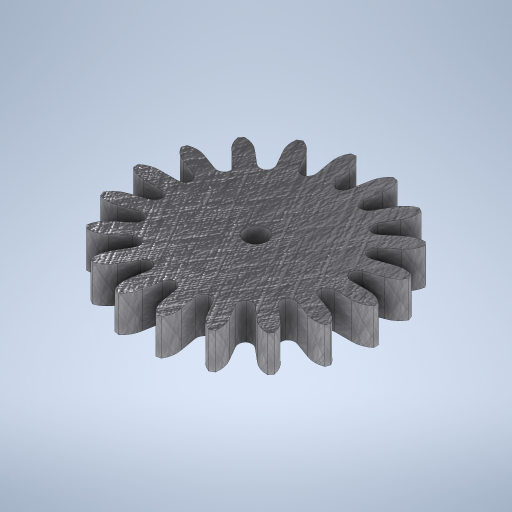
# Autodesk Inventor part: Rear_motor
Saved by Autodesk Inventor 2024 (Build 280153020, 153B)
## iProperties
Created: 2023-05-21
Part Number: Rear_motor
Material: Generic
Document SubType Name: Modeling
Designer: Diego
Density: 1 g/cm^3
Appearance: Default
Author: Diego
Autodesk Inventor part; units mm, degrees
ref_plane "YZ Plane" through (0, 0, 0) normal (1, 0, 0) x (0, 1, 0)
ref_plane "XZ Plane" through (0, 0, 0) normal (0, 1, 0) x (-1, 0, 0)
ref_plane "XY Plane" through (0, 0, 0) normal (0, 0, 1) x (1, 0, 0)
sketch "Sketch1" plane through (0, 0, 0) normal (0, 1, 0) x (-1, 0, 0)
  circle A0 centre (0, 0) radius 1.4
  arc A1 (14.997, -0.3) -> (14.997, 0.3) centre (0, 0) ccw
  line L0 (0, 0) -> (19.0442, 1.4988) construction
  line L1 (0, 0) -> (19.3478, 0) construction
  line L2 (0, 0) -> (18.7398, -1.4749) construction
  arc A2 (14.997, 0.3) -> (12.9599, 1.02) centre (13.0458, -1.9788) ccw
  arc A3 (12.9599, -1.02) -> (14.997, -0.3) centre (13.0458, 1.9788) ccw
  line L3 (12.9599, 1.02) -> (10.8129, 1.02)
  line L4 (12.9599, -1.02) -> (10.8129, -1.02)
  arc A4 (10.8129, -1.02) -> (9.8299, -1.8363) centre (10.8129, -2.02) ccw
  arc A5 (9.8299, 1.8363) -> (10.8129, 1.02) centre (10.8129, 2.02) ccw
  line L5 (12.5272, 3.4741) -> (10.5097, 2.7398)
  arc A6 (10.5097, 2.7398) -> (9.8652, 1.6364) centre (10.8517, 1.8001) ccw
  arc A7 (8.6091, 5.0876) -> (9.812, 4.6567) centre (9.47, 5.5964) ccw
  arc A8 (13.99, 5.4112) -> (11.8295, 5.391) centre (12.9359, 2.6025) ccw
  line L6 (11.8295, 5.391) -> (9.812, 4.6567)
  arc A9 (14.1952, 4.8474) -> (13.99, 5.4112) centre (0, 0) ccw
  arc A10 (12.5272, 3.4741) -> (14.1952, 4.8474) centre (11.5823, 6.3214) ccw
  line L7 (10.5835, 7.5491) -> (8.9388, 6.1691)
  arc A11 (8.9388, 6.1691) -> (8.7106, 4.9119) centre (9.5816, 5.403) ccw
  arc A12 (6.3498, 7.7253) -> (7.6276, 7.7318) centre (6.9848, 8.4978) ccw
  arc A13 (11.2955, 9.8697) -> (9.2723, 9.1118) centre (11.2656, 6.8698) ccw
  line L8 (9.2723, 9.1118) -> (7.6276, 7.7318)
  arc A14 (11.6812, 9.4101) -> (11.2955, 9.8697) centre (0, 0) ccw
  arc A15 (10.5835, 7.5491) -> (11.6812, 9.4101) centre (8.7217, 9.9015) ccw
  line L9 (7.3633, 10.7136) -> (6.2898, 8.8543)
  arc A16 (6.2898, 8.8543) -> (6.5053, 7.5948) centre (7.1558, 8.3543) ccw
  arc A17 (3.3247, 9.4312) -> (4.5232, 9.8743) centre (3.6571, 10.3743) ccw
  arc A18 (7.2387, 13.1378) -> (5.5966, 11.7336) centre (8.2366, 10.3086) ccw
  line L10 (5.5966, 11.7336) -> (4.5232, 9.8743)
  arc A19 (7.7583, 12.8378) -> (7.2387, 13.1378) centre (0, 0) ccw
  arc A20 (7.3633, 10.7136) -> (7.7583, 12.8378) centre (4.8092, 12.2874) ccw
  line L11 (3.2549, 12.5859) -> (2.8821, 10.4716)
  arc A21 (2.8821, 10.4716) -> (3.5154, 9.3617) centre (3.8669, 10.2979) ccw
  arc A22 (-0.1015, 9.9995) -> (0.8732, 10.8258) centre (-0.1116, 10.9994) ccw
  arc A23 (2.3088, 14.8213) -> (1.246, 12.9402) centre (4.2141, 12.504) ccw
  line L12 (1.246, 12.9402) -> (0.8732, 10.8258)
  arc A24 (2.8996, 14.7171) -> (2.3088, 14.8213) centre (0, 0) ccw
  arc A25 (3.2549, 12.5859) -> (2.8996, 14.7171) centre (0.3166, 13.1912) ccw
  line L13 (-1.246, 12.9402) -> (-0.8732, 10.8258)
  arc A26 (-0.8732, 10.8258) -> (0.1015, 9.9995) centre (0.1116, 10.9994) ccw
  arc A27 (-3.5154, 9.3617) -> (-2.8821, 10.4716) centre (-3.8669, 10.2979) ccw
  arc A28 (-2.8996, 14.7171) -> (-3.2549, 12.5859) centre (-0.3166, 13.1912) ccw
  line L14 (-3.2549, 12.5859) -> (-2.8821, 10.4716)
  arc A29 (-2.3088, 14.8213) -> (-2.8996, 14.7171) centre (0, 0) ccw
  arc A30 (-1.246, 12.9402) -> (-2.3088, 14.8213) centre (-4.2141, 12.504) ccw
  line L15 (-5.5966, 11.7336) -> (-4.5232, 9.8743)
  arc A31 (-4.5232, 9.8743) -> (-3.3247, 9.4312) centre (-3.6571, 10.3743) ccw
  arc A32 (-6.5053, 7.5948) -> (-6.2898, 8.8543) centre (-7.1558, 8.3543) ccw
  arc A33 (-7.7583, 12.8378) -> (-7.3633, 10.7136) centre (-4.8092, 12.2874) ccw
  line L16 (-7.3633, 10.7136) -> (-6.2898, 8.8543)
  arc A34 (-7.2387, 13.1378) -> (-7.7583, 12.8378) centre (0, 0) ccw
  arc A35 (-5.5966, 11.7336) -> (-7.2387, 13.1378) centre (-8.2366, 10.3086) ccw
  line L17 (-9.2723, 9.1118) -> (-7.6276, 7.7318)
  arc A36 (-7.6276, 7.7318) -> (-6.3498, 7.7253) centre (-6.9848, 8.4978) ccw
  arc A37 (-8.7106, 4.9119) -> (-8.9388, 6.1691) centre (-9.5816, 5.403) ccw
  arc A38 (-11.6812, 9.4101) -> (-10.5835, 7.5491) centre (-8.7217, 9.9015) ccw
  line L18 (-10.5835, 7.5491) -> (-8.9388, 6.1691)
  arc A39 (-11.2955, 9.8697) -> (-11.6812, 9.4101) centre (0, 0) ccw
  arc A40 (-9.2723, 9.1118) -> (-11.2955, 9.8697) centre (-11.2656, 6.8698) ccw
  line L19 (-11.8295, 5.391) -> (-9.812, 4.6567)
  arc A41 (-9.812, 4.6567) -> (-8.6091, 5.0876) centre (-9.47, 5.5964) ccw
  arc A42 (-9.8652, 1.6364) -> (-10.5097, 2.7398) centre (-10.8517, 1.8001) ccw
  arc A43 (-14.1952, 4.8474) -> (-12.5272, 3.4741) centre (-11.5823, 6.3214) ccw
  line L20 (-12.5272, 3.4741) -> (-10.5097, 2.7398)
  arc A44 (-13.99, 5.4112) -> (-14.1952, 4.8474) centre (0, 0) ccw
  arc A45 (-11.8295, 5.391) -> (-13.99, 5.4112) centre (-12.9359, 2.6025) ccw
  line L21 (-12.9599, 1.02) -> (-10.8129, 1.02)
  arc A46 (-10.8129, 1.02) -> (-9.8299, 1.8363) centre (-10.8129, 2.02) ccw
  arc A47 (-9.8299, -1.8363) -> (-10.8129, -1.02) centre (-10.8129, -2.02) ccw
  arc A48 (-14.997, -0.3) -> (-12.9599, -1.02) centre (-13.0458, 1.9788) ccw
  line L22 (-12.9599, -1.02) -> (-10.8129, -1.02)
  arc A49 (-14.997, 0.3) -> (-14.997, -0.3) centre (0, 0) ccw
  arc A50 (-12.9599, 1.02) -> (-14.997, 0.3) centre (-13.0458, -1.9788) ccw
  line L23 (-12.5272, -3.4741) -> (-10.5097, -2.7398)
  arc A51 (-10.5097, -2.7398) -> (-9.8652, -1.6364) centre (-10.8517, -1.8001) ccw
  arc A52 (-8.6091, -5.0876) -> (-9.812, -4.6567) centre (-9.47, -5.5964) ccw
  arc A53 (-13.99, -5.4112) -> (-11.8295, -5.391) centre (-12.9359, -2.6025) ccw
  line L24 (-11.8295, -5.391) -> (-9.812, -4.6567)
  arc A54 (-14.1952, -4.8474) -> (-13.99, -5.4112) centre (0, 0) ccw
  arc A55 (-12.5272, -3.4741) -> (-14.1952, -4.8474) centre (-11.5823, -6.3214) ccw
  line L25 (-10.5835, -7.5491) -> (-8.9388, -6.1691)
  arc A56 (-8.9388, -6.1691) -> (-8.7106, -4.9119) centre (-9.5816, -5.403) ccw
  arc A57 (-6.3498, -7.7253) -> (-7.6276, -7.7318) centre (-6.9848, -8.4978) ccw
  arc A58 (-11.2955, -9.8697) -> (-9.2723, -9.1118) centre (-11.2656, -6.8698) ccw
  line L26 (-9.2723, -9.1118) -> (-7.6276, -7.7318)
  arc A59 (-11.6812, -9.4101) -> (-11.2955, -9.8697) centre (0, 0) ccw
  arc A60 (-10.5835, -7.5491) -> (-11.6812, -9.4101) centre (-8.7217, -9.9015) ccw
  line L27 (-7.3633, -10.7136) -> (-6.2898, -8.8543)
  arc A61 (-6.2898, -8.8543) -> (-6.5053, -7.5948) centre (-7.1558, -8.3543) ccw
  arc A62 (-3.3247, -9.4312) -> (-4.5232, -9.8743) centre (-3.6571, -10.3743) ccw
  arc A63 (-7.2387, -13.1378) -> (-5.5966, -11.7336) centre (-8.2366, -10.3086) ccw
  line L28 (-5.5966, -11.7336) -> (-4.5232, -9.8743)
  arc A64 (-7.7583, -12.8378) -> (-7.2387, -13.1378) centre (0, 0) ccw
  arc A65 (-7.3633, -10.7136) -> (-7.7583, -12.8378) centre (-4.8092, -12.2874) ccw
  line L29 (-3.2549, -12.5859) -> (-2.8821, -10.4716)
  arc A66 (-2.8821, -10.4716) -> (-3.5154, -9.3617) centre (-3.8669, -10.2979) ccw
  arc A67 (0.1015, -9.9995) -> (-0.8732, -10.8258) centre (0.1116, -10.9994) ccw
  arc A68 (-2.3088, -14.8213) -> (-1.246, -12.9402) centre (-4.2141, -12.504) ccw
  line L30 (-1.246, -12.9402) -> (-0.8732, -10.8258)
  arc A69 (-2.8996, -14.7171) -> (-2.3088, -14.8213) centre (0, 0) ccw
  arc A70 (-3.2549, -12.5859) -> (-2.8996, -14.7171) centre (-0.3166, -13.1912) ccw
  line L31 (1.246, -12.9402) -> (0.8732, -10.8258)
  arc A71 (0.8732, -10.8258) -> (-0.1015, -9.9995) centre (-0.1116, -10.9994) ccw
  arc A72 (3.5154, -9.3617) -> (2.8821, -10.4716) centre (3.8669, -10.2979) ccw
  arc A73 (2.8996, -14.7171) -> (3.2549, -12.5859) centre (0.3166, -13.1912) ccw
  line L32 (3.2549, -12.5859) -> (2.8821, -10.4716)
  arc A74 (2.3088, -14.8213) -> (2.8996, -14.7171) centre (0, 0) ccw
  arc A75 (1.246, -12.9402) -> (2.3088, -14.8213) centre (4.2141, -12.504) ccw
  line L33 (5.5966, -11.7336) -> (4.5232, -9.8743)
  arc A76 (4.5232, -9.8743) -> (3.3247, -9.4312) centre (3.6571, -10.3743) ccw
  arc A77 (6.5053, -7.5948) -> (6.2898, -8.8543) centre (7.1558, -8.3543) ccw
  arc A78 (7.7583, -12.8378) -> (7.3633, -10.7136) centre (4.8092, -12.2874) ccw
  line L34 (7.3633, -10.7136) -> (6.2898, -8.8543)
  arc A79 (7.2387, -13.1378) -> (7.7583, -12.8378) centre (0, 0) ccw
  arc A80 (5.5966, -11.7336) -> (7.2387, -13.1378) centre (8.2366, -10.3086) ccw
  line L35 (9.2723, -9.1118) -> (7.6276, -7.7318)
  arc A81 (7.6276, -7.7318) -> (6.3498, -7.7253) centre (6.9848, -8.4978) ccw
  arc A82 (8.7106, -4.9119) -> (8.9388, -6.1691) centre (9.5816, -5.403) ccw
  arc A83 (11.6812, -9.4101) -> (10.5835, -7.5491) centre (8.7217, -9.9015) ccw
  line L36 (10.5835, -7.5491) -> (8.9388, -6.1691)
  arc A84 (11.2955, -9.8697) -> (11.6812, -9.4101) centre (0, 0) ccw
  arc A85 (9.2723, -9.1118) -> (11.2955, -9.8697) centre (11.2656, -6.8698) ccw
  line L37 (11.8295, -5.391) -> (9.812, -4.6567)
  arc A86 (9.812, -4.6567) -> (8.6091, -5.0876) centre (9.47, -5.5964) ccw
  arc A87 (9.8652, -1.6364) -> (10.5097, -2.7398) centre (10.8517, -1.8001) ccw
  arc A88 (14.1952, -4.8474) -> (12.5272, -3.4741) centre (11.5823, -6.3214) ccw
  line L38 (12.5272, -3.4741) -> (10.5097, -2.7398)
  arc A89 (13.99, -5.4112) -> (14.1952, -4.8474) centre (0, 0) ccw
  arc A90 (11.8295, -5.391) -> (13.99, -5.4112) centre (12.9359, -2.6025) ccw
  arc A91 (8.7106, 4.9119) -> (8.6091, 5.0876) centre (0, 0) ccw
  arc A92 (6.5053, 7.5948) -> (6.3498, 7.7253) centre (0, 0) ccw
  arc A93 (3.5154, 9.3617) -> (3.3247, 9.4312) centre (0, 0) ccw
  arc A94 (0.1015, 9.9995) -> (-0.1015, 9.9995) centre (0, 0) ccw
  arc A95 (-3.3247, 9.4312) -> (-3.5154, 9.3617) centre (0, 0) ccw
  arc A96 (-6.3498, 7.7253) -> (-6.5053, 7.5948) centre (0, 0) ccw
  arc A97 (-8.6091, 5.0876) -> (-8.7106, 4.9119) centre (0, 0) ccw
  arc A98 (-9.8299, 1.8363) -> (-9.8652, 1.6364) centre (0, 0) ccw
  arc A99 (-9.8652, -1.6364) -> (-9.8299, -1.8363) centre (0, 0) ccw
  arc A100 (-8.7106, -4.9119) -> (-8.6091, -5.0876) centre (0, 0) ccw
  arc A101 (-6.5053, -7.5948) -> (-6.3498, -7.7253) centre (0, 0) ccw
  arc A102 (-3.5154, -9.3617) -> (-3.3247, -9.4312) centre (0, 0) ccw
  arc A103 (-0.1015, -9.9995) -> (0.1015, -9.9995) centre (0, 0) ccw
  arc A104 (3.3247, -9.4312) -> (3.5154, -9.3617) centre (0, 0) ccw
  arc A105 (6.3498, -7.7253) -> (6.5053, -7.5948) centre (0, 0) ccw
  arc A106 (8.6091, -5.0876) -> (8.7106, -4.9119) centre (0, 0) ccw
  circle A107 centre (0, 0) radius 10 construction
  circle A108 centre (0, 0) radius 13.0054 construction
  circle A109 centre (0, 0) radius 15 construction
  point P0 (9.9478, -1.02)
  point P1 (9.9478, 1.02)
  point P2 (9.8537, 1.7375)
  point P3 (8.6652, 5.0028)
  point P4 (6.4315, 7.6648)
  point P5 (3.4221, 9.4023)
  point P6 (0, 10.0057)
  point P7 (-3.4221, 9.4023)
  point P8 (-6.4315, 7.6648)
  point P9 (-8.6652, 5.0028)
  point P10 (-9.8537, 1.7375)
  point P11 (-9.8537, -1.7375)
  point P12 (-8.6652, -5.0028)
  point P13 (-6.4315, -7.6648)
  point P14 (-3.4221, -9.4023)
  point P15 (0, -10.0057)
  point P16 (3.4221, -9.4023)
  point P17 (6.4315, -7.6648)
  point P18 (8.6652, -5.0028)
  point P19 (9.8537, -1.7375)
  dimension "d0" = 2.8
  dimension "d4" = 9
  dimension "d5" = 4.5
  dimension "d6" = 3
  dimension "d7" = 0.3
  dimension "d8" = 0.6
  dimension "d9" = 3
  dimension "d11" = 1
  dimension "d12" = 1
  dimension "d15" = 360
  dimension "d19" = 20
  constraints: 212 point on circle, 110 centre point, 78 end point, 5 coincident, 4 point on line, 3 horizontal, 2 tangent, 361 other
  measures "d0" diameter of A0
  measures "d4" angle of L2 L0
  measures "d5" angle of L2 L1
  measures "d6" radius of A2
  measures "d7" distance from line of L1 A1.end
  measures "d8" distance of A1.end A1.start
  measures "d9" radius of A3
  measures "d11" radius of A4
  measures "d12" radius of A5
  measures "d19" diameter of A107
extrude "Extrusion1" add sketch "Sketch1" along normal blind 4.5
body "Solid1"
